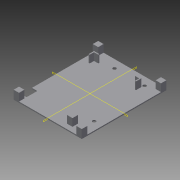
# Autodesk Inventor part: sensor3
Saved by Autodesk Inventor 2015 SP2 (Build 190223200, 223)
## iProperties
Created: 2016-02-10
Part Number: sensor3
Material: Generic
Document SubType Name: Modeling
Designer: mca20
Density: 1 g/cm^3
Appearance: Default
Author: mca20
Autodesk Inventor part; units mm, degrees
ref_plane "YZ Plane" through (0, 0, 0) normal (1, 0, 0) x (0, 1, 0)
ref_plane "XZ Plane" through (0, 0, 0) normal (0, 1, 0) x (-1, 0, 0)
ref_plane "XY Plane" through (0, 0, 0) normal (0, 0, 1) x (1, 0, 0)
sketch "Sketch1" plane through (0, 0, 0) normal (0, 1, 0) x (-1, 0, 0)
  line L0 (0, 0) -> (53.34, 0)
  line L1 (53.34, 0) -> (53.34, -68.58)
  line L2 (53.34, -68.58) -> (0, -68.58)
  line L3 (0, -68.58) -> (0, 0)
  line L4 (53.34, -66) -> (0, -66) construction
  circle A0 centre (7.62, -66) radius 1.5
  circle A1 centre (35.56, -66) radius 1.5
  circle A2 centre (2.5, -14) radius 1.5
  line L5 (-5, -73.58) -> (58.34, -73.58)
  line L6 (58.34, -73.58) -> (58.34, 5)
  line L7 (58.34, 5) -> (-5, 5)
  line L8 (-5, 5) -> (-5, -73.58)
  dimension "d0" = 68.58
  dimension "d1" = 53.34
  dimension "d2" = 2.58
  dimension "d3" = 3
  dimension "d4" = 7.62
  dimension "d5" = 3
  dimension "d6" = 35.56
  dimension "d8" = 3
  dimension "d9" = 14
  dimension "d10" = 2.5
  dimension "d46" = 5
  dimension "d73" = 63.34
  dimension "d74" = 78.58
  constraints: 18 end point, 4 parallel, 4 point on line, 3 centre point, 3 perpendicular, 1 horizontal, 3 other
  measures "d0" distance between parallel lines of L2 L0
  measures "d1" distance between parallel lines of L3 L1
  measures "d2" distance between parallel lines of L2 L4
  measures "d3" diameter of A0
  measures "d4" distance from line of L3 A0.centre
  measures "d5" diameter of A1
  measures "d6" distance from line of L3 A1.centre
  measures "d8" diameter of A2
  measures "d9" distance from line of L0 A2.centre
  measures "d10" distance from line of L3 A2.centre
  measures "d46" distance between parallel lines of L2 L5
  measures "d73" distance between parallel lines of L8 L6
  measures "d74" distance between parallel lines of L7 L5
extrude "Extrusion4" add sketch "Sketch1" along normal blind 1 contours L0 L1 L2 L3 | L8 L7 L6 L5
sketch "Sketch5" plane through (0, 1, 0) normal (0, 1, 0) x (1, 0, 0)
  line L0 (5, -5) -> (0, -5)
  line L1 (0, -5) -> (0, 0)
  line L2 (0, 0) -> (5, 0)
  line L3 (5, 0) -> (5, -5)
  dimension "d49" = 5
  dimension "d50" = 5
  constraints: 8 end point, 2 parallel, 1 horizontal, 1 perpendicular
  measures "d49" distance of L1.end L2.end
  measures "d50" distance of L0.end L1.end
extrude "Extrusion5" add sketch "Sketch5" along normal blind 7
ref_plane "Work Plane2" through (-26.67, 0, 5) normal (1, 0, 0) x (0, 0, -1)
mirror "Mirror2" about plane through (-26.67, 0, 5) normal (1, 0, 0) of "Extrusion5"
ref_plane "Work Plane3" through (-58.34, 0, -34.29) normal (0, 0, 1) x (1, 0, 0)
mirror "Mirror3" about plane through (-58.34, 0, -34.29) normal (0, 0, 1) of "Extrusion5", "Mirror2"
sketch "Sketch6" plane through (0, 1, 0) normal (0, 1, 0) x (1, 0, 0)
  line L0 (-51.17, 0.5) -> (-9.17, 0.5)
  line L1 (-9.17, 0.5) -> (-9.17, 62.5)
  line L2 (-9.17, 62.5) -> (-51.17, 62.5)
  line L3 (-51.17, 62.5) -> (-51.17, 0.5)
  line L4 (-52.17, 63.5) -> (-8.17, 63.5)
  line L5 (-8.17, 63.5) -> (-8.17, -0.5)
  line L6 (-8.17, -0.5) -> (-52.17, -0.5)
  line L7 (-52.17, -0.5) -> (-52.17, 63.5)
  line L8 (-52.17, 4.5) -> (-51.17, 4.5)
  line L9 (-47.17, 0.5) -> (-47.17, -0.5)
  line L10 (-47.17, 63.5) -> (-47.17, 62.5)
  line L11 (-51.17, 58.5) -> (-52.17, 58.5)
  line L12 (-13.17, 0.5) -> (-13.17, -0.5)
  line L13 (-9.17, 4.5) -> (-8.17, 4.5)
  line L14 (-9.17, 58.5) -> (-8.17, 58.5)
  line L15 (-13.17, 63.5) -> (-13.17, 62.5)
  point P0 (0, 0)
  point P1 (-30.17, 0.5)
  dimension "d34" = 42
  dimension "d35" = 62
  dimension "d39" = 1
  dimension "d40" = 5
  dimension "d41" = 5
  dimension "d44" = 5
  dimension "d45" = 5
  dimension "d62" = 5
  dimension "d63" = 5
  dimension "d64" = 5
  dimension "d65" = 5
  constraints: 32 end point, 16 point on line, 10 perpendicular, 4 parallel, 1 horizontal, 1 midpoint, 3 other
  measures "d34" distance of L2.end L1.end
  measures "d35" distance of L1.end L0.end
  measures "d39" distance between parallel lines of L2 L4
  measures "d40" distance between parallel lines of L6 L8
  measures "d41" distance from line of L7 L9.end
  measures "d44" distance from line of L11.end L4
  measures "d45" distance between parallel lines of L7 L10
  measures "d62" distance between parallel lines of L15 L5
  measures "d63" distance between parallel lines of L14 L4
  measures "d64" distance between parallel lines of L5 L12
  measures "d65" distance between parallel lines of L6 L13
sketch "Sketch7" plane through (0, 8, 0) normal (0, 1, 0) x (1, 0, 0)
  line L0 (0, 0) -> (0, -5) projected
  line L1 (0, -5) -> (5, -5) projected
  line L2 (5, -5) -> (5, 0) projected
  line L3 (5, 0) -> (0, 0) projected
  circle A0 centre (2.5, -2.5) radius 1
  dimension "d53" = 5
  dimension "d54" = 2
  constraints: 1 centre point
  measures "d53" distance between parallel lines of L1 L3
  measures "d54" diameter of A0
hole "Hole1" [suppressed]
mirror "Mirror8" [suppressed]
mirror "Mirror9" [suppressed]
extrude "Extrusion8" add sketch "Sketch6" along normal blind 7 contours L0 L1 L13 L5 L6 L12 | L11 L7 L4 L10 L2 L3 | L1 L2 L15 L4 L5 L14
sketch "Sketch8" plane through (0, 1, 0) normal (0, 1, 0) x (1, 0, 0)
  line L0 (-58.34, 73.58) -> (-58.34, -5) projected
  line L1 (-58.34, 2) -> (-53.34, 2)
  line L2 (-53.34, 2) -> (-53.34, 12)
  line L3 (-53.34, 12) -> (-58.34, 12)
  line L4 (-58.34, 12) -> (-58.34, 2)
  line L5 (-58.34, 0) -> (-53.34, 0) projected
  point P0 (0, 0)
  dimension "d68" = 5
  dimension "d69" = 10
  dimension "d70" = 2
  constraints: 8 end point, 2 parallel, 1 horizontal, 1 perpendicular, 1 point on line
  measures "d68" distance of L3.end L2.end
  measures "d69" distance of L2.end L1.end
  measures "d70" distance between parallel lines of L1 L5
extrude "Extrusion9" cut sketch "Sketch8" against normal blind 1
body "Solid2"
body "Solid3"
